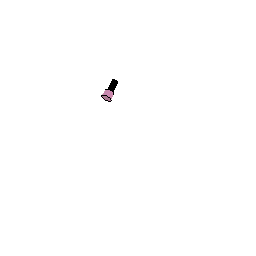
screw (Autodesk Fusion 360 design; units mm, degrees)
Autodesk Fusion 360 part; units mm, degrees
note: some values were not read from the file. Set by a fixed rule: which face or edge a step refers to.
sketch "Sketch1" plane through (14.6619, -51.9135, -54.4721) normal (0.243103, -0.860756, -0.447214) x (0.962354, 0.271798, 0)
  circle A0 centre (-0.6326, 50.893) radius 2
  dimension "d353" = 0
  dimension "d354" = 0
  dimension "d355" = 0
  dimension "d356" = 0
  dimension "d365" = 0
  dimension "d366" = 0
  dimension "d367" = 0
  dimension "d368" = 0
  dimension "d377" = 0
  dimension "d378" = 0
  dimension "d379" = 0
  dimension "d380" = 0
  dimension "d413" = 0
  dimension "d414" = 0
  dimension "d415" = 0
  dimension "d416" = 0
  dimension "d425" = 0
  dimension "d426" = 0
  dimension "d427" = 0
  dimension "d428" = 0
  dimension "d437" = 0
  dimension "d438" = 0
  dimension "d439" = 0
  dimension "d440" = 0
  dimension "d449" = 0
  dimension "d450" = 0
  dimension "d451" = 0
  dimension "d452" = 0
  dimension "d461" = 0
  dimension "d462" = 0
  dimension "d463" = 0
  dimension "d464" = 0
  dimension "d473" = 0
  dimension "d474" = 0
  dimension "d475" = 0
  dimension "d476" = 0
  dimension "d485" = 0
  dimension "d486" = 0
  dimension "d487" = 0
  dimension "d488" = 0
  dimension "d493" = 0
  dimension "d494" = 0
  dimension "d495" = 0
  dimension "d496" = 0
  dimension "d505" = 0
  dimension "d506" = 0
  dimension "d507" = 0
  dimension "d508" = 0
  dimension "d517" = 0
  dimension "d518" = 0
  dimension "d519" = 0
  dimension "d520" = 0
  dimension "d534" = 4
  dimension "d535" = 0
  dimension "d536" = 0
  dimension "d537" = 0
  dimension "d538" = 0
  dimension "d543" = 0
  dimension "d544" = 0
  dimension "d545" = 0
  dimension "d546" = 0
  measures "d534" diameter of A0
extrude "Extrude1" add sketch "Sketch1" along normal blind 0.2 and the other way blind 8 makes body 1
sketch "Sketch2" plane through (17.7003, -62.6716, -32.5616) normal (0.243103, -0.860756, -0.447214) x (0.962354, 0.271798, 0)
  circle A0 centre (-0.6326, 26.2963) radius 3
  ellipse E0 centre (-0.6326, 26.2963) end of major axis (-0.6359, 24.2963) minor radius 2
  circle A1 centre (-0.6326, 26.2963) radius 2
  dimension "d338" = 6
  constraint concentric A0 E0
  measures "d338" diameter of A0
extrude "Extrude2" add sketch "Sketch2" along normal blind 5 draft 5 separate body contours A0 | E0 A1 makes body 2
thread "Thread1" "ISO Metric profile 4.0 M4x0.7 6g" major diameter 3.908 minor diameter 3.111 pitch 0.7 angle 60 modelled right hand crest width 0.1017 on face at (21.7275, -74.3892, -7.6704) crest through (20.1323, -66.4209, -5.296) on face at (20.3985, -69.6837, -5.2256) crest through (20.1323, -66.4209, -5.296) on bodies 1
